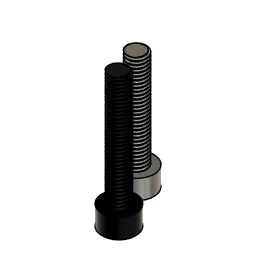
Стенд v5 (Autodesk Fusion 360 archive; units mm, degrees)
design "M6 Hex Screw v3"
Autodesk Fusion 360 part; units mm, degrees
sketch "Sketch1" plane through (0, 0, 0) normal (0, 0, 1) x (1, 0, 0)
  line L0 (0, 0) -> (15, 0) construction
  circle A0 centre (15, 0) radius 5.11
  dimension "d1" = 15
  dimension "d2" = 10.22
  constraint coincident L0.start origin
  constraint horizontal L0
  constraint coincident L0.end A0.centre
  measures "d1" distance of L0.start L0.end
  measures "d2" diameter of A0
extrude "Extrude1" add sketch "Sketch1" along normal blind 6 makes body 1
sketch "Sketch2" plane through (0, 0, 0) normal (0, 0, -1) x (1, 0, 0)
  circle A0 centre (15, 0) radius 5.11
  line L0 (12.43, -1.4838) -> (15, -2.9676)
  line L1 (15, -2.9676) -> (17.57, -1.4838)
  line L2 (17.57, -1.4838) -> (17.57, 1.4838)
  line L3 (17.57, 1.4838) -> (15, 2.9676)
  line L4 (15, 2.9676) -> (12.43, 1.4838)
  line L5 (12.43, 1.4838) -> (12.43, -1.4838)
  point P0 (15, 0)
  dimension "d5" = 2.57
  constraint coincident P0 A0.centre
  constraint vertical L5
  measures "d5" distance of P0 L5
extrude "Extrude2" cut sketch "Sketch2" against normal blind 3 contours L0 L1 L2 L3 L4 L5 bodies 1
fillet "Fillet1" radius 0.2 1 edges at (10.2358, -1.8479, 0) on bodies 1
pattern_circular "C-Pattern1" count 6 over 360 about axis through (0, 0, 1.75) along (0, 0, 1) of bodies 1 makes body 2 at (10.2724, 17.2829, 4.0667) makes body 3 at (-9.8312, 17.5376, 4.0667) makes body 4 at (-20.1036, 0.2547, 4.0667) makes body 5 at (-10.2724, -17.2829, 4.0667) makes body 6 at (9.8312, -17.5376, 4.0667)
sketch "Sketch3" plane through (0, 0, 6) normal (0, 0, 1) x (-1, 0, 0)
  circle A0 centre (-15, 0) radius 5.11
  circle A1 centre (-7.5, -12.9904) radius 5.11
  circle A2 centre (7.5, -12.9904) radius 5.11
  circle A3 centre (15, 0) radius 5.11
  circle A4 centre (7.5, 12.9904) radius 5.11
  circle A5 centre (-7.5, 12.9904) radius 5.11
  circle A6 centre (-15, 0) radius 3
  circle A7 centre (-7.5, -12.9904) radius 3
  circle A8 centre (7.5, -12.9904) radius 3
  circle A9 centre (15, 0) radius 3
  circle A10 centre (7.5, 12.9904) radius 3
  circle A11 centre (-7.5, 12.9904) radius 3
  dimension "d12" = 6
  constraint concentric A0 A6
  constraint concentric A1 A7
  constraint concentric A2 A8
  constraint concentric A3 A9
  constraint concentric A4 A10
  constraint concentric A5 A11
  constraint equal A6 A7
  constraint equal A7 A8
  constraint equal A8 A9
  constraint equal A9 A10
  constraint equal A10 A11
  measures "d12" diameter of A6
extrude "Extrude3" add sketch "Sketch3" along normal blind 10 contours A11 bodies 6
extrude "Extrude4" add sketch "Sketch3" along normal blind 15 contours A6 bodies 1
extrude "Extrude5" add sketch "Sketch3" along normal blind 20 contours A7 bodies 2
extrude "Extrude6" add sketch "Sketch3" along normal blind 25 contours A8 bodies 3
extrude "Extrude7" add sketch "Sketch3" along normal blind 30 contours A9 bodies 4
extrude "Extrude8" add sketch "Sketch3" along normal blind 35 contours A10 bodies 5
thread "Thread1" "ISO Metric profile 6.0 M6x1 6g" major diameter 5.884 minor diameter 4.7435 pitch 1 angle 60 modelled right hand crest width 0.1444 on face at (12.0149, 0.2987, 16) crest through (12.058, 0, 5.75) on face at (-10.4851, 13.2891, 14.3333) crest through (-10.442, 12.9904, 5.75) on face at (-17.9851, 0.2987, 26) crest through (-17.942, 0, 5.75) on face at (-10.4851, -12.6917, 29.3333) crest through (-10.442, -12.9904, 5.75) on face at (4.5037, -12.8408, 12.6667) crest through (4.558, -12.9904, 5.75) on face at (4.5037, 13.1399, 19.3333) crest through (4.558, 12.9904, 5.75) on bodies 1 2 3 4 5 6
hidden bodies 1 2 3 6

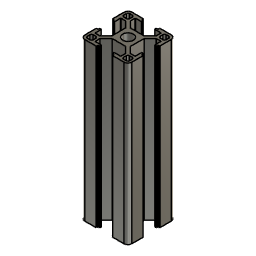
design "profilo alluminio 3030_100mm"
Autodesk Fusion 360 part; units mm, degrees
sketch "Schizzo1" plane through (0, 0, 0) normal (0, 0, 1) x (1, 0, 0)
  circle A0 centre (0, 4) radius 3.4
  line L0 (-12.5, 17.5) -> (-10.7, 17.5) construction
  line L1 (-12.5, 17.5) -> (-10.7, 17.5)
  line L2 (-9.7, 16.5) -> (-9.7, 14.7)
  line L3 (-10.7, 13.7) -> (-12.5, 13.7)
  line L4 (-13.5, 14.7) -> (-13.5, 16.5)
  arc A1 (-9.7, 16.5) -> (-10.7, 17.5) centre (-10.7, 16.5) ccw
  arc A2 (-10.7, 13.7) -> (-9.7, 14.7) centre (-10.7, 14.7) ccw
  arc A3 (-13.5, 14.7) -> (-12.5, 13.7) centre (-12.5, 14.7) ccw
  arc A4 (-12.5, 17.5) -> (-13.5, 16.5) centre (-12.5, 16.5) ccw
  arc A5 (-12.5, 19) -> (-15, 16.5) centre (-12.5, 16.5) ccw
  line L5 (0, 22) -> (0, -17) construction
  line L6 (-9.7, 16.5) -> (-9.7, 19.7766) construction
  line L7 (-12.5, 19) -> (-9.7, 19)
  line L8 (-9.7, 19) -> (-8.2, 19)
  line L9 (-12.8, 12) -> (-12.8, 8.33)
  line L10 (-15, 16.5) -> (-15, 12.2)
  line L11 (-15, 12.2) -> (-15, 9.43)
  line L12 (-13.9, 8.87) -> (-13.9, 8.33)
  line L13 (-13.62, 8.05) -> (-13.08, 8.05)
  line L14 (-12.6, 12.2) -> (-9.816, 12.2)
  line L15 (-9.618, 12.118) -> (-5.882, 8.382)
  line L16 (-8.2, 19) -> (-5.35, 19)
  line L17 (-5.15, 18.8) -> (-5.15, 18.18)
  line L18 (-4.87, 17.9) -> (-4.33, 17.9)
  line L19 (-4.05, 17.62) -> (-4.05, 17.08)
  line L20 (-4.33, 16.8) -> (-7.92, 16.8)
  line L21 (-8.2, 16.52) -> (-8.2, 13.816)
  line L22 (-8.118, 13.618) -> (-4.3003, 9.8003)
  line L23 (0, 4) -> (-21.8842, 3.95)
  line L24 (0, 21) -> (0, -20)
  line L25 (-14.18, 9.15) -> (-14.8, 9.15)
  line L26 (-15, 9.35) -> (-15, 9.43)
  line L27 (-13.9, 8.87) -> (-13.9, 8.95)
  line L28 (-14.1, 9.15) -> (-14.18, 9.15)
  line L29 (-13.9, 8.33) -> (-13.9, 8.25)
  line L30 (-13.7, 8.05) -> (-13.62, 8.05)
  line L31 (-12.8, 8.25) -> (-12.8, 8.33)
  line L32 (-13.08, 8.05) -> (-13, 8.05)
  line L33 (-9.618, 12.118) -> (-9.6414, 12.1414)
  line L34 (-9.7828, 12.2) -> (-9.816, 12.2)
  line L35 (-4.87, 17.9) -> (-4.95, 17.9)
  line L36 (-5.15, 18.18) -> (-5.15, 18.1)
  line L37 (-4.33, 17.9) -> (-4.25, 17.9)
  line L38 (-4.05, 17.7) -> (-4.05, 17.62)
  line L39 (-4.05, 17.08) -> (-4.05, 17)
  line L40 (-4.25, 16.8) -> (-4.33, 16.8)
  line L41 (-7.92, 16.8) -> (-8, 16.8)
  line L42 (-8.2, 16.6) -> (-8.2, 16.52)
  arc A6 (-15, 9.35) -> (-14.8, 9.15) centre (-14.8, 9.35) ccw
  arc A7 (-13.9, 8.95) -> (-14.1, 9.15) centre (-14.1, 8.95) ccw
  arc A8 (-13.9, 8.25) -> (-13.7, 8.05) centre (-13.7, 8.25) ccw
  arc A9 (-13, 8.05) -> (-12.8, 8.25) centre (-13, 8.25) ccw
  arc A10 (-12.6, 12.2) -> (-12.8, 12) centre (-12.6, 12) ccw
  arc A11 (-9.6414, 12.1414) -> (-9.7828, 12.2) centre (-9.7828, 12) ccw
  line L43 (-8.2, 13.816) -> (-8.2, 13.7)
  line L44 (-8.2, 13.7) -> (-8.118, 13.618)
  arc A12 (-5.15, 18.8) -> (-5.35, 19) centre (-5.35, 18.8) ccw
  arc A13 (-5.15, 18.1) -> (-4.95, 17.9) centre (-4.95, 18.1) ccw
  arc A14 (-4.05, 17.7) -> (-4.25, 17.9) centre (-4.25, 17.7) ccw
  arc A15 (-4.25, 16.8) -> (-4.05, 17) centre (-4.25, 17) ccw
  arc A16 (-8, 16.8) -> (-8.2, 16.6) centre (-8, 16.6) ccw
  line L45 (-4.2664, -9.9196) -> (-4.1864, -9.9193)
  line L46 (-8.074, -5.655) -> (-4.2738, -1.8199)
  line L47 (-4.2715, -8.8197) -> (-7.8614, -8.8361)
  line L48 (-3.9902, -9.0984) -> (-3.9906, -9.0184)
  line L49 (-4.1915, -8.8193) -> (-4.2715, -8.8197)
  line L50 (-4.8064, -9.9221) -> (-4.2664, -9.9196)
  line L51 (-12.7633, -4.0584) -> (-12.7801, -0.3884)
  line L52 (-14.9754, -1.4185) -> (-14.975, -1.4985)
  line L53 (-12.7804, -0.3084) -> (-12.7801, -0.3884)
  arc A17 (-14.0763, -1.2144) -> (-13.8772, -1.0135) centre (-14.0772, -1.0144) ccw
  line L54 (-9.6314, -11.0442) -> (-8.1314, -11.0373)
  line L55 (-9.5808, -4.1619) -> (-9.6041, -4.1854)
  line L56 (-9.7453, -4.2446) -> (-9.7784, -4.2448)
  arc A18 (-8.1423, -8.6373) -> (-7.9414, -8.8364) centre (-7.9423, -8.6364) ccw
  line L57 (-4.8064, -9.9221) -> (-4.8864, -9.9225)
  line L58 (-12.4382, -9.557) -> (-10.6382, -9.5488)
  arc A19 (-14.9427, -8.5684) -> (-12.4313, -11.057) centre (-12.4428, -8.557) ccw
  arc A20 (-9.651, -6.7442) -> (-10.6556, -5.7488) centre (-10.651, -6.7488) ccw
  line L59 (-9.5808, -4.1619) -> (-5.8619, -0.4088)
  arc A21 (-12.4555, -5.757) -> (-13.451, -6.7616) centre (-12.451, -6.757) ccw
  line L60 (-13.8776, -0.9335) -> (-13.8772, -1.0135)
  arc A22 (-5.2814, -11.0243) -> (-5.0823, -10.8234) centre (-5.2823, -10.8243) ccw
  arc A23 (-12.7804, -0.3084) -> (-12.9814, -0.1094) centre (-12.9804, -0.3094) ccw
  line L61 (-14.9624, -4.2685) -> (-14.975, -1.4985)
  line L62 (-13.8801, -0.3935) -> (-13.8804, -0.3135)
  line L63 (-12.5624, -4.2575) -> (-9.7784, -4.2448)
  arc A24 (-13.4427, -8.5616) -> (-12.4382, -9.557) centre (-12.4428, -8.557) ccw
  line L64 (-14.0763, -1.2144) -> (-14.1563, -1.2147)
  line L65 (-5.0852, -10.2034) -> (-5.0855, -10.1234)
  line L66 (-8.1551, -5.8533) -> (-8.1556, -5.7374)
  line L67 (-9.6428, -8.5442) -> (-9.6278, -11.8208) construction
  line L68 (-12.4313, -11.057) -> (-9.6314, -11.0442)
  line L69 (-8.1423, -8.6373) -> (-8.1427, -8.5573)
  arc A25 (-9.7453, -4.2446) -> (-9.6041, -4.1854) centre (-9.7462, -4.0446) ccw
  line L70 (-7.8614, -8.8361) -> (-7.9414, -8.8364)
  line L71 (-8.1427, -8.5573) -> (-8.1551, -5.8533)
  line L72 (-10.6556, -5.7488) -> (-12.4555, -5.757)
  line L73 (-13.451, -6.7616) -> (-13.4427, -8.5616)
  arc A26 (-4.8864, -9.9225) -> (-5.0855, -10.1234) centre (-4.8855, -10.1225) ccw
  line L74 (-8.1314, -11.0373) -> (-5.2814, -11.0243)
  line L75 (-8.1556, -5.7374) -> (-8.074, -5.655)
  line L76 (-13.8776, -0.9335) -> (-13.8801, -0.3935)
  line L77 (-13.6014, -0.1122) -> (-13.0614, -0.1097)
  line L78 (-13.0614, -0.1097) -> (-12.9814, -0.1094)
  arc A27 (-10.6382, -9.5488) -> (-9.6428, -8.5442) centre (-10.6428, -8.5488) ccw
  line L79 (-9.6428, -8.5442) -> (-9.651, -6.7442)
  arc A28 (-13.6814, -0.1126) -> (-13.8804, -0.3135) centre (-13.6804, -0.3126) ccw
  line L80 (-14.1563, -1.2147) -> (-14.7763, -1.2176)
  arc A29 (-3.9906, -9.0184) -> (-4.1915, -8.8193) centre (-4.1906, -9.0193) ccw
  line L81 (-14.9427, -8.5684) -> (-14.9624, -4.2685)
  line L82 (-3.9874, -9.7184) -> (-3.9877, -9.6384)
  line L83 (-13.6814, -0.1126) -> (-13.6014, -0.1122)
  arc A30 (-12.7633, -4.0584) -> (-12.5624, -4.2575) centre (-12.5633, -4.0575) ccw
  line L84 (-5.0823, -10.8234) -> (-5.0852, -10.2034)
  arc A31 (-4.1864, -9.9193) -> (-3.9874, -9.7184) centre (-4.1874, -9.7193) ccw
  line L85 (-3.9877, -9.6384) -> (-3.9902, -9.0984)
  arc A32 (-14.7763, -1.2176) -> (-14.9754, -1.4185) centre (-14.7754, -1.4176) ccw
  line L86 (-12.4382, -9.557) -> (-10.6382, -9.5488) construction
  line L87 (-5.882, 8.382) -> (-5.8619, -0.4088)
  line L88 (4.33, 16.8) -> (7.92, 16.8)
  line L89 (4.87, 17.9) -> (4.33, 17.9)
  line L90 (8.074, -5.655) -> (4.2738, -1.8199)
  arc A33 (4.25, 17.9) -> (4.05, 17.7) centre (4.25, 17.7) ccw
  line L91 (4.25, 16.8) -> (4.33, 16.8)
  line L92 (4.05, 17.7) -> (4.05, 17.62)
  arc A34 (13.451, -6.7616) -> (12.4555, -5.757) centre (12.451, -6.757) ccw
  line L93 (5.0852, -10.2034) -> (5.0855, -10.1234)
  line L94 (9.7453, -4.2446) -> (9.7784, -4.2448)
  line L95 (8.1551, -5.8533) -> (8.1556, -5.7374)
  line L96 (9.7, 16.5) -> (9.7, 14.7)
  line L97 (9.6428, -8.5442) -> (9.651, -6.7442)
  line L98 (5.15, 18.8) -> (5.15, 18.18)
  line L99 (14.9427, -8.5684) -> (14.9624, -4.2685)
  line L100 (10.7, 13.7) -> (12.5, 13.7)
  arc A35 (5.35, 19) -> (5.15, 18.8) centre (5.35, 18.8) ccw
  line L101 (7.92, 16.8) -> (8, 16.8)
  line L102 (8.2, 13.816) -> (8.2, 13.7)
  arc A36 (12.5624, -4.2575) -> (12.7633, -4.0584) centre (12.5633, -4.0575) ccw
  arc A37 (10.6556, -5.7488) -> (9.651, -6.7442) centre (10.651, -6.7488) ccw
  line L103 (8.118, 13.618) -> (4.3003, 9.8003)
  line L104 (4.05, 17.08) -> (4.05, 17)
  line L105 (7.8614, -8.8361) -> (7.9414, -8.8364)
  line L106 (12.4382, -9.557) -> (10.6382, -9.5488)
  line L107 (13.6014, -0.1122) -> (13.0614, -0.1097)
  arc A38 (12.9814, -0.1094) -> (12.7804, -0.3084) centre (12.9804, -0.3094) ccw
  line L108 (14.1563, -1.2147) -> (14.7763, -1.2176)
  line L109 (4.8064, -9.9221) -> (4.2664, -9.9196)
  arc A39 (13.8804, -0.3135) -> (13.6814, -0.1126) centre (13.6804, -0.3126) ccw
  line L110 (13.0614, -0.1097) -> (12.9814, -0.1094)
  line L111 (9.7828, 12.2) -> (9.816, 12.2)
  line L112 (14.0763, -1.2144) -> (14.1563, -1.2147)
  arc A40 (7.9414, -8.8364) -> (8.1423, -8.6373) centre (7.9423, -8.6364) ccw
  arc A41 (12.4382, -9.557) -> (13.4427, -8.5616) centre (12.4428, -8.557) ccw
  line L113 (15, 9.35) -> (15, 9.43)
  line L114 (13.8776, -0.9335) -> (13.8772, -1.0135)
  line L115 (9.6428, -8.5442) -> (9.6278, -11.8208) construction
  line L116 (13.5, 14.7) -> (13.5, 16.5)
  line L117 (9.618, 12.118) -> (5.882, 8.382)
  line L118 (13.6814, -0.1126) -> (13.6014, -0.1122)
  line L119 (8.1556, -5.7374) -> (8.074, -5.655)
  arc A42 (14.9754, -1.4185) -> (14.7763, -1.2176) centre (14.7754, -1.4176) ccw
  line L120 (8.2, 16.52) -> (8.2, 13.816)
  arc A43 (13.8772, -1.0135) -> (14.0763, -1.2144) centre (14.0772, -1.0144) ccw
  line L121 (12.8, 12) -> (12.8, 8.33)
  line L122 (3.9877, -9.6384) -> (3.9902, -9.0984)
  arc A44 (3.9874, -9.7184) -> (4.1864, -9.9193) centre (4.1874, -9.7193) ccw
  line L123 (4.1915, -8.8193) -> (4.2715, -8.8197)
  line L124 (5.882, 8.382) -> (5.8619, -0.4088)
  arc A45 (4.1915, -8.8193) -> (3.9906, -9.0184) centre (4.1906, -9.0193) ccw
  line L125 (14.9624, -4.2685) -> (14.975, -1.4985)
  line L126 (9.5808, -4.1619) -> (5.8619, -0.4088)
  arc A46 (4.05, 17) -> (4.25, 16.8) centre (4.25, 17) ccw
  line L127 (4.05, 17.62) -> (4.05, 17.08)
  line L128 (4.33, 17.9) -> (4.25, 17.9)
  line L129 (4.2715, -8.8197) -> (7.8614, -8.8361)
  line L130 (4.8064, -9.9221) -> (4.8864, -9.9225)
  line L131 (13.9, 8.33) -> (13.9, 8.25)
  line L132 (8.2, 13.7) -> (8.118, 13.618)
  line L133 (12.5, 19) -> (9.7, 19)
  arc A47 (5.0855, -10.1234) -> (4.8864, -9.9225) centre (4.8855, -10.1225) ccw
  arc A48 (14.1, 9.15) -> (13.9, 8.95) centre (14.1, 8.95) ccw
  line L134 (12.5624, -4.2575) -> (9.7784, -4.2448)
  line L135 (13.62, 8.05) -> (13.08, 8.05)
  line L136 (8.1427, -8.5573) -> (8.1551, -5.8533)
  line L137 (9.7, 19) -> (8.2, 19)
  line L138 (12.6, 12.2) -> (9.816, 12.2)
  arc A49 (10.7, 17.5) -> (9.7, 16.5) centre (10.7, 16.5) ccw
  line L139 (12.8, 8.25) -> (12.8, 8.33)
  line L140 (10.6556, -5.7488) -> (12.4555, -5.757)
  line L141 (13.08, 8.05) -> (13, 8.05)
  arc A50 (9.6428, -8.5442) -> (10.6382, -9.5488) centre (10.6428, -8.5488) ccw
  arc A51 (9.7828, 12.2) -> (9.6414, 12.1414) centre (9.7828, 12) ccw
  line L142 (13.7, 8.05) -> (13.62, 8.05)
  line L143 (9.7, 16.5) -> (9.7, 19.7766) construction
  arc A52 (15, 16.5) -> (12.5, 19) centre (12.5, 16.5) ccw
  line L144 (8.2, 16.6) -> (8.2, 16.52)
  line L145 (5.0823, -10.8234) -> (5.0852, -10.2034)
  line L146 (13.8776, -0.9335) -> (13.8801, -0.3935)
  arc A53 (13.5, 16.5) -> (12.5, 17.5) centre (12.5, 16.5) ccw
  arc A54 (9.6041, -4.1854) -> (9.7453, -4.2446) centre (9.7462, -4.0446) ccw
  line L147 (13.9, 8.87) -> (13.9, 8.33)
  line L148 (8.1423, -8.6373) -> (8.1427, -8.5573)
  arc A55 (9.7, 14.7) -> (10.7, 13.7) centre (10.7, 14.7) ccw
  arc A56 (12.8, 12) -> (12.6, 12.2) centre (12.6, 12) ccw
  line L149 (9.6314, -11.0442) -> (8.1314, -11.0373)
  arc A57 (12.4313, -11.057) -> (14.9427, -8.5684) centre (12.4428, -8.557) ccw
  line L150 (8.2, 19) -> (5.35, 19)
  arc A58 (4.95, 17.9) -> (5.15, 18.1) centre (4.95, 18.1) ccw
  arc A59 (12.5, 13.7) -> (13.5, 14.7) centre (12.5, 14.7) ccw
  line L151 (9.5808, -4.1619) -> (9.6041, -4.1854)
  line L152 (14.1, 9.15) -> (14.18, 9.15)
  line L153 (9.618, 12.118) -> (9.6414, 12.1414)
  line L154 (12.7804, -0.3084) -> (12.7801, -0.3884)
  line L155 (5.15, 18.18) -> (5.15, 18.1)
  line L156 (13.451, -6.7616) -> (13.4427, -8.5616)
  line L157 (12.4382, -9.557) -> (10.6382, -9.5488) construction
  arc A60 (14.8, 9.15) -> (15, 9.35) centre (14.8, 9.35) ccw
  arc A61 (8.2, 16.6) -> (8, 16.8) centre (8, 16.6) ccw
  line L158 (12.5, 17.5) -> (10.7, 17.5)
  line L159 (13.8801, -0.3935) -> (13.8804, -0.3135)
  line L160 (14.9754, -1.4185) -> (14.975, -1.4985)
  line L161 (4.87, 17.9) -> (4.95, 17.9)
  line L162 (8.1314, -11.0373) -> (5.2814, -11.0243)
  line L163 (14.18, 9.15) -> (14.8, 9.15)
  arc A62 (5.0823, -10.8234) -> (5.2814, -11.0243) centre (5.2823, -10.8243) ccw
  line L164 (12.4313, -11.057) -> (9.6314, -11.0442)
  arc A63 (13.7, 8.05) -> (13.9, 8.25) centre (13.7, 8.25) ccw
  arc A64 (12.8, 8.25) -> (13, 8.05) centre (13, 8.25) ccw
  line L165 (3.9874, -9.7184) -> (3.9877, -9.6384)
  line L166 (15, 12.2) -> (15, 9.43)
  line L167 (13.9, 8.87) -> (13.9, 8.95)
  line L168 (3.9902, -9.0984) -> (3.9906, -9.0184)
  line L169 (15, 16.5) -> (15, 12.2)
  line L170 (12.5, 17.5) -> (10.7, 17.5) construction
  line L171 (12.7633, -4.0584) -> (12.7801, -0.3884)
  line L172 (4.2664, -9.9196) -> (4.1864, -9.9193)
  line L173 (-4.3003, 9.8003) -> (4.3003, 9.8003)
  line L174 (-4.2738, -1.8199) -> (4.2738, -1.8199)
  point P0 (-15, 19)
  point P1 (-13.5, 13.7)
  point P2 (-12.8, 8.05)
  point P3 (-13.9, 9.15)
  point P4 (-13.9, 8.05)
  point P5 (-9.7, 12.2)
  point P6 (-5.15, 19)
  point P7 (-5.15, 17.9)
  point P8 (-4.05, 17.9)
  point P9 (-4.05, 16.8)
  point P10 (-8.2, 16.8)
  point P11 (-15, 9.15)
  point P12 (-13.8813, -0.1135)
  point P13 (-14.9313, -11.0684)
  point P14 (-5.0814, -11.0234)
  point P15 (-13.4555, -5.7616)
  point P16 (-13.8763, -1.2135)
  point P17 (-8.1414, -8.8373)
  point P18 (-12.7814, -0.1084)
  point P19 (-3.9864, -9.9184)
  point P20 (-3.9915, -8.8184)
  point P21 (-14.9763, -1.2185)
  point P22 (-5.0864, -9.9234)
  point P23 (-9.6624, -4.2442)
  point P24 (3.9915, -8.8184)
  point P25 (15, 9.15)
  point P26 (12.8, 8.05)
  point P27 (15, 19)
  point P28 (13.4555, -5.7616)
  point P29 (13.8763, -1.2135)
  point P30 (8.1414, -8.8373)
  point P31 (5.15, 19)
  point P32 (9.6624, -4.2442)
  point P33 (3.9864, -9.9184)
  point P34 (5.0864, -9.9234)
  point P35 (13.9, 9.15)
  point P36 (9.7, 12.2)
  point P37 (4.05, 17.9)
  point P38 (13.8813, -0.1135)
  point P39 (14.9313, -11.0684)
  point P40 (8.2, 16.8)
  point P41 (13.5, 13.7)
  point P42 (14.9763, -1.2185)
  point P43 (13.9, 8.05)
  point P44 (12.7814, -0.1084)
  point P45 (5.0814, -11.0234)
  point P46 (4.05, 16.8)
  point P47 (5.15, 17.9)
  dimension "d1" = 6.8
  dimension "d2" = 1
  dimension "d3" = 1
  dimension "d4" = 2.5
  dimension "d5" = 1.5
  dimension "d6" = 3.05
  dimension "d7" = 1.1
  dimension "d8" = 1.1
  dimension "d9" = 1.1
  dimension "d10" = 4.15
  dimension "d11" = 2.77
  dimension "d12" = 0.28
  dimension "d13" = 0.2
  dimension "d14" = 0.2
  dimension "d15" = 0.2
  constraint horizontal L0
  constraint horizontal L1
  constraint vertical L2
  constraint horizontal L3
  constraint vertical L4
  constraint tangent L2 A1
  constraint tangent L0 A1
  constraint tangent L2 A2
  constraint tangent L3 A2
  constraint equal A1 A2
  constraint coincident P1 L3
  constraint coincident P1 L4
  constraint tangent L3 A3
  constraint tangent L4 A3
  constraint equal A1 A3
  constraint tangent L0 A4
  constraint tangent A1 L6
  constraint coincident L6 L7.end
  constraint tangent A5 L7
  constraint perpendicular L6 L7
  constraint perpendicular L6 L8
  constraint tangent A5 L10
  constraint parallel L8 L16
  constraint perpendicular L16 L17
  constraint perpendicular L17 L18
  constraint perpendicular L16 L19
  constraint perpendicular L19 L20
  constraint perpendicular L16 L21
  constraint coincident A0.centre L23.start
  constraint coincident P4 L12
  constraint coincident P4 L13
  constraint coincident P3 L12
  constraint coincident P2 L13
  constraint coincident P2 L9
  constraint coincident P5 L14
  constraint coincident P5 L15
  constraint coincident P10 L21
  constraint coincident P10 L20
  constraint coincident P9 L20
  constraint coincident P9 L19
  constraint coincident P8 L19
  constraint coincident P8 L18
  constraint coincident P7 L17
  constraint coincident P7 L18
  constraint coincident L5 L24.start
  constraint perpendicular L11 L25
  constraint perpendicular L25 L26
  constraint perpendicular L25 L29
  constraint perpendicular L29 L30
  constraint perpendicular L13 L31
  constraint perpendicular L31 L32
  constraint parallel L14 L34
  constraint parallel L16 L35
  constraint perpendicular L35 L36
  constraint perpendicular L36 L37
  constraint perpendicular L37 L38
  constraint perpendicular L37 L39
  constraint perpendicular L39 L40
  constraint perpendicular L39 L41
  constraint perpendicular L41 L42
  constraint coincident P11 L25
  constraint coincident P11 L26
  constraint tangent L25 A6
  constraint tangent L26 A6
  constraint tangent L27 A7
  constraint tangent L28 A7
  constraint equal A6 A7
  constraint tangent L29 A8
  constraint tangent L30 A8
  constraint equal A6 A8
  constraint tangent L32 A9
  constraint tangent L31 A9
  constraint equal A6 A9
  constraint tangent L9 A10
  constraint tangent L14 A10
  constraint equal A6 A10
  constraint tangent L34 A11
  constraint tangent L33 A11
  constraint parallel L21 L43
  constraint parallel L22 L44
  constraint coincident P6 L16
  constraint coincident P6 L17
  constraint tangent L16 A12
  constraint tangent L17 A12
  constraint tangent L35 A13
  constraint tangent L36 A13
  constraint equal A12 A13
  constraint tangent L37 A14
  constraint tangent L38 A14
  constraint equal A12 A14
  constraint tangent L39 A15
  constraint tangent L40 A15
  constraint equal A12 A15
  constraint tangent L41 A16
  constraint tangent L42 A16
  constraint equal A12 A16
  constraint symmetric P0 L23 P13
  constraint symmetric P1 L23 P15
  constraint symmetric L2.start L23 L67.start
  constraint symmetric L0.end L23 L58.end
  constraint symmetric A1 L23 A27
  constraint symmetric L2.end L23 A20.start
  constraint symmetric L3.start L23 A20.end
  constraint symmetric A2 L23 A20
  constraint symmetric L3.end L23 A21.start
  constraint symmetric L4.start L23 A21.end
  constraint symmetric A3 L23 A21
  constraint symmetric L0.start L23 L58.start
  constraint symmetric L4.end L23 A24.start
  constraint symmetric A4 L23 A24
  constraint symmetric A5.start L23 A19.end
  constraint symmetric A5.end L23 A19.start
  constraint symmetric A5 L23 A19
  constraint symmetric L6.end L23 L67.end
  constraint symmetric L7.end L23 L54.start
  constraint symmetric L8.end L23 L54.end
  constraint symmetric L10.end L23 L61.start
  constraint symmetric P2 L23 P18
  constraint symmetric P3 L23 P16
  constraint symmetric P4 L23 P12
  constraint symmetric P5 L23 P23
  constraint symmetric P6 L23 P14
  constraint symmetric P7 L23 P22
  constraint symmetric P8 L23 P19
  constraint symmetric P9 L23 P20
  constraint symmetric P10 L23 P17
  constraint symmetric L22.end L23 L46.end
  constraint symmetric L23 L11.end L52.end
  constraint symmetric L23 L12.end L62.start
  constraint symmetric L23 L13.start L77.start
  constraint symmetric L23 L25.start L64.end
  constraint symmetric L23 L12.start L60.start
  constraint symmetric L23 L13.end L77.end
  constraint symmetric L23 L9.end L51.end
  constraint symmetric L23 L14.end L56.end
  constraint symmetric L23 L15.start L55.start
  constraint symmetric L23 L15.end L59.end
  constraint symmetric L23 L22.start L46.start
  constraint symmetric L23 L21.end L66.start
  constraint symmetric L23 L21.start L69.end
  constraint symmetric L23 L20.end L47.end
  constraint symmetric L23 L20.start L47.start
  constraint symmetric L23 L19.end L48.start
  constraint symmetric L23 L19.start L82.end
  constraint symmetric L23 L18.end L45.start
  constraint symmetric L23 L17.end L65.start
  constraint symmetric L23 L18.start L50.start
  constraint symmetric L23 P11 P21
  constraint symmetric L23 L25.end L80.end
  constraint symmetric L23 L26.start L52.start
  constraint symmetric L23 A6 A32
  constraint symmetric L23 L27.end A17.end
  constraint symmetric L23 L28.start A17.start
  constraint symmetric L23 A7 A17
  constraint symmetric L23 L29.end L62.end
  constraint symmetric L23 L30.start A28.start
  constraint symmetric L23 A8 A28
  constraint symmetric L23 L32.end A23.end
  constraint symmetric L23 L31.start L53.start
  constraint symmetric L23 A9 A23
  constraint symmetric L23 L9.start L51.start
  constraint symmetric L23 L14.start L63.start
  constraint symmetric L23 A10 A30
  constraint symmetric L23 L34.start L56.start
  constraint symmetric L23 L33.end L55.end
  constraint symmetric L23 A11 A25
  constraint symmetric L23 L43.end L66.end
  constraint symmetric L23 L16.end A22.start
  constraint symmetric L23 L17.start A22.end
  constraint symmetric L23 A12 A22
  constraint symmetric L23 L35.end L57.end
  constraint symmetric L23 L36.end L65.end
  constraint symmetric L23 A13 A26
  constraint symmetric L23 L37.end L45.end
  constraint symmetric L23 L38.start L82.start
  constraint symmetric L23 A14 A31
  constraint symmetric L23 L39.end L48.end
  constraint symmetric L23 L40.start L49.start
  constraint symmetric L23 A15 A29
  constraint symmetric L23 L41.end A18.end
  constraint symmetric L23 L42.start A18.start
  constraint symmetric L23 A16 A18
  constraint symmetric P0 L24 P27
  constraint symmetric P1 L24 P41
  constraint symmetric L2.start L24 L96.start
  constraint symmetric L0.end L24 A49.start
  constraint symmetric A1 L24 A49
  constraint symmetric L2.end L24 L96.end
  constraint symmetric L3.start L24 L100.start
  constraint symmetric A2 L24 A55
  constraint symmetric L3.end L24 L100.end
  constraint symmetric L4.start L24 L116.start
  constraint symmetric A3 L24 A59
  constraint symmetric L0.start L24 A53.end
  constraint symmetric L4.end L24 L116.end
  constraint symmetric A4 L24 A53
  constraint symmetric A5.start L24 L133.start
  constraint symmetric A5.end L24 A52.start
  constraint symmetric A5 L24 A52
  constraint symmetric L6.end L24 L143.end
  constraint symmetric L7.end L24 L133.end
  constraint symmetric L8.end L24 L137.end
  constraint symmetric L10.end L24 L166.start
  constraint symmetric P2 L24 P26
  constraint symmetric P3 L24 P35
  constraint symmetric P4 L24 P43
  constraint symmetric P5 L24 P36
  constraint symmetric P6 L24 P31
  constraint symmetric P7 L24 P47
  constraint symmetric P8 L24 P37
  constraint symmetric P9 L24 P46
  constraint symmetric P10 L24 P40
  constraint symmetric L22.end L24 L103.end
  constraint symmetric L11.end L24 L113.end
  constraint symmetric L12.end L24 L131.start
  constraint symmetric L13.start L24 L135.start
  constraint symmetric L25.start L24 L152.end
  constraint symmetric L12.start L24 L147.start
  constraint symmetric L13.end L24 L135.end
  constraint symmetric L9.end L24 L121.end
  constraint symmetric L14.end L24 L111.end
  constraint symmetric L15.start L24 L117.start
  constraint symmetric L15.end L24 L117.end
  constraint symmetric L22.start L24 L103.start
  constraint symmetric L21.end L24 L102.start
  constraint symmetric L21.start L24 L120.start
  constraint symmetric L20.end L24 L88.end
  constraint symmetric L20.start L24 L88.start
  constraint symmetric L19.end L24 L104.start
  constraint symmetric L19.start L24 L92.end
  constraint symmetric L18.end L24 L89.end
  constraint symmetric L17.end L24 L98.end
  constraint symmetric L18.start L24 L89.start
  constraint symmetric L24 P11 P25
  constraint symmetric L24 L25.end A60.start
  constraint symmetric L24 L26.start L113.start
  constraint symmetric L24 A6 A60
  constraint symmetric L24 L27.end A48.end
  constraint symmetric L24 L28.start A48.start
  constraint symmetric L24 A7 A48
  constraint symmetric L24 L29.end L131.end
  constraint symmetric L24 L30.start L142.start
  constraint symmetric L24 A8 A63
  constraint symmetric L24 L32.end L141.end
  constraint symmetric L24 L31.start L139.start
  constraint symmetric L24 A9 A64
  constraint symmetric L24 L9.start L121.start
  constraint symmetric L24 L14.start L138.start
  constraint symmetric L24 A10 A56
  constraint symmetric L24 L34.start L111.start
  constraint symmetric L24 L33.end A51.end
  constraint symmetric L24 A11 A51
  constraint symmetric L24 L43.end L102.end
  constraint symmetric L24 L16.end A35.start
  constraint symmetric L24 L17.start L98.start
  constraint symmetric L24 A12 A35
  constraint symmetric L24 L35.end A58.start
  constraint symmetric L24 L36.end A58.end
  constraint symmetric L24 A13 A58
  constraint symmetric L24 L37.end A33.start
  constraint symmetric L24 L38.start A33.end
  constraint symmetric L24 A14 A33
  constraint symmetric L24 L39.end L104.end
  constraint symmetric L24 L40.start L91.start
  constraint symmetric L24 A15 A46
  constraint symmetric L24 L41.end L101.end
  constraint symmetric L24 L42.start L144.start
  constraint symmetric L24 A16 A61
  constraint symmetric L24 L65.end L93.end
  constraint symmetric L24 L50.start L109.start
  constraint symmetric L24 L48.end A45.end
  constraint symmetric L24 L45.end A44.end
  constraint symmetric L24 A20.start L97.end
  constraint symmetric L24 A22.end L145.start
  constraint symmetric L24 L65.start L93.start
  constraint symmetric L24 A22.start L162.end
  constraint symmetric L24 A20.end A37.start
  constraint symmetric L24 L66.end L95.end
  constraint symmetric L24 L77.start L107.start
  constraint symmetric L24 L64.end L108.start
  constraint symmetric L24 L57.end L130.end
  constraint symmetric L24 L60.start L114.start
  constraint symmetric L24 L49.start L123.start
  constraint symmetric L24 L82.start A44.start
  constraint symmetric L24 P12 P38
  constraint symmetric L24 L62.end A39.start
  constraint symmetric L24 L53.start A38.end
  constraint symmetric L24 L51.end L154.end
  constraint symmetric L24 L62.start L146.end
  constraint symmetric L24 A28.start A39.end
  constraint symmetric L24 L47.start L123.end
  constraint symmetric L24 A17.end L114.end
  constraint symmetric L24 A17.start L112.start
  constraint symmetric L24 L52.end L125.end
  constraint symmetric L24 L67.start L97.start
  constraint symmetric L24 L48.start L122.end
  constraint symmetric L24 A23.end A38.start
  constraint symmetric L24 L82.end L122.start
  constraint symmetric L24 L80.end L108.end
  constraint symmetric L24 L77.end L107.end
  constraint symmetric L24 L45.start L109.end
  constraint symmetric L24 L58.end L106.end
  constraint symmetric L24 L52.start A42.start
  constraint symmetric L24 L67.end L115.end
  constraint symmetric L24 P13 P39
  constraint symmetric L24 L51.start A36.end
  constraint symmetric L24 L54.end L149.end
  constraint symmetric L24 A19.start L99.start
  constraint symmetric L24 P14 P45
  constraint symmetric L24 L66.start L95.start
  constraint symmetric L24 L46.start L90.start
  constraint symmetric L24 A18.start A40.end
  constraint symmetric L24 A24.start A41.end
  constraint symmetric L24 L55.start L126.start
  constraint symmetric L24 P15 P28
  constraint symmetric L24 L56.start L94.start
  constraint symmetric L24 A21.end A34.start
  constraint symmetric L24 L69.end L136.start
  constraint symmetric L24 P16 P29
  constraint symmetric L24 P17 P30
  constraint symmetric L24 L54.start L149.start
  constraint symmetric L24 L59.end L124.end
  constraint symmetric L24 L46.end L90.end
  constraint symmetric L24 A19.end A57.start
  constraint symmetric L24 P18 P44
  constraint symmetric L24 L61.start L99.end
  constraint symmetric L24 P19 P33
  constraint symmetric L24 A18.end L105.end
  constraint symmetric L24 L47.end L105.start
  constraint symmetric L24 P20 P24
  constraint symmetric L24 P21 P42
  constraint symmetric L24 P22 P34
  constraint symmetric L24 A21.start A34.end
  constraint symmetric L24 L56.end L94.end
  constraint symmetric L24 L58.start L106.start
  constraint symmetric L24 L63.start A36.start
  constraint symmetric L24 P23 P32
  constraint symmetric L24 L55.end A54.start
  constraint symmetric L24 A17 A43
  constraint symmetric L24 A18 A40
  constraint symmetric L24 A19 A57
  constraint symmetric L24 A20 A37
  constraint symmetric L24 A21 A34
  constraint symmetric L24 A22 A62
  constraint symmetric L24 A23 A38
  constraint symmetric L24 A24 A41
  constraint symmetric L24 A25 A54
  constraint symmetric L24 A26 A47
  constraint symmetric L24 A27 A50
  constraint symmetric L24 A28 A39
  constraint symmetric L24 A29 A45
  constraint symmetric L24 A30 A36
  constraint symmetric L24 A31 A44
  constraint symmetric L24 A32 A42
  measures "d1" diameter of A0
  measures "d2" radius of A1
  measures "d3" radius of A4
  measures "d4" radius of A5
  measures "d5" distance of L7.end L8.end
  measures "d6" distance of L8.end P6
  measures "d7" distance of P6 P7
  measures "d8" distance of P7 P8
  measures "d9" distance of P8 P9
  measures "d10" distance of P9 P10
  measures "d11" distance of L10.end L11.end
  measures "d12" distance of L11.end P11
  measures "d13" radius of A6
  measures "d14" radius of A11
  measures "d15" radius of A12
extrude "Estrusione1" add sketch "Schizzo1" along normal blind 100 contours A0 L24 L88 L89 L90 A33 L91 L92 L93 L94 L95 L98 L99 A35 L101 L102 A36 L103 L104 L105 L107 A38 L108 L109 A39 L110 L111 L112 A40 L113 L114 L117 L118 L119 A42 L120 A43 L121 L122 A44 L123 L124 A45 L125 L126 A46 L127 L128 L129 L130 L131 L132 L133 A47 A48 L134 L135 L136 L137 L138 L139 L141 A51 L142 A52 L144 L145 L146 A54 L147 L148 A56 L149 A57 L150 A58 L151 L152 L153 L154 L155 A60 A61 L159 L160 L161 L162 L163 A62 L164 A63 A64 L165 L166 L167 L168 L169 L171 L172 L173 L174 | A0 A5 L7 L8 L9 L10 L11 L12 L13 L14 L15 L16 L17 L18 L19 L20 L21 L22 L23 L24 L25 L26 L27 L28 L29 L30 L31 L32 L33 L34 L35 L36 L37 L38 L39 L40 L41 L42 A6 A7 A8 A9 A10 A11 L43 L44 A12 A13 A14 A15 A16 L87 L173 | A0 L23 L24 L45 L46 L47 L48 L49 L50 L51 L52 L53 A17 L54 L55 L56 A18 L57 A19 L59 L60 A22 A23 L61 L62 L63 L64 L65 L66 L68 L69 A25 L70 L71 A26 L74 L75 L76 L77 L78 A28 L80 A29 L81 L82 L83 A30 L84 A31 L85 A32 L87 L174

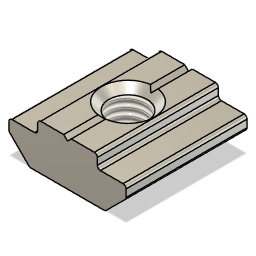
design "Slider T-Nut for 3030 - M6"
Autodesk Fusion 360 part; units mm, degrees
sketch "Sketch1" plane through (0, 0, 0) normal (0, 0, 1) x (1, 0, 0)
  line L0 (2.0362, -0.8565) -> (12.0362, -0.8565)
  line L1 (14.7862, 1.8935) -> (14.7862, 3.4435)
  line L2 (-0.7138, 3.4435) -> (-0.7138, 1.8935)
  line L3 (10.9862, 3.4435) -> (10.9862, 5.1435)
  line L4 (3.0862, 5.1435) -> (3.0862, 3.4435)
  line L5 (-0.7138, 1.8935) -> (2.0362, -0.8565)
  line L6 (7.8157, 5.425) -> (7.8157, -0.8565) construction
  line L7 (14.7862, 1.8935) -> (12.0362, -0.8565)
  line L8 (14.7862, 3.4435) -> (10.9862, 3.4435)
  line L9 (3.0862, 3.4435) -> (-0.7138, 3.4435)
  line L10 (7.0362, 4.6435) -> (7.5362, 5.1435)
  line L11 (7.0362, 4.6435) -> (9.6302, 4.6435) construction
  line L12 (7.0362, 4.6435) -> (6.5362, 5.1435)
  line L13 (7.0362, 4.6435) -> (9.6237, 4.6435) construction
  line L14 (10.9862, 5.1435) -> (7.5362, 5.1435)
  line L15 (6.5362, 5.1435) -> (3.0862, 5.1435)
  dimension "d10" = 3.8
  dimension "d12" = 45
  dimension "d26" = 15.5
  dimension "d27" = 6
  dimension "d28" = 7.9
  dimension "d30" = 7.75
  dimension "d32" = 3.8
  dimension "d33" = 0.5
  dimension "d34" = 1.7
  dimension "d35" = 10
  dimension "d36" = 135
  dimension "d37" = 135
  dimension "d38" = 2.75
  dimension "d39" = 2.75
  constraint horizontal L0
  constraint vertical L1
  constraint horizontal L8
  constraint vertical L2
  constraint vertical L3
  constraint horizontal L14
  constraint vertical L4
  constraint coincident L4.end L8
  constraint coincident L0 L6.end
  constraint perpendicular L0 L6
  constraint collinear L8 L9
  constraint horizontal L11
  constraint perpendicular L10 L12
  constraint horizontal L13
  constraint collinear L14 L15
  constraint equal L1 L2
  constraint equal L5 L7
  measures "d10" distance of L1.end L3.start
  measures "d12" angle of L10 L11
  measures "d26" distance of L1 L2
  measures "d27" distance of L0 L15
  measures "d28" distance of L3 L4
  measures "d30" distance of L2 L10.start
  measures "d32" distance of L2 L4
  measures "d33" distance of L10.start L15
  measures "d34" distance of L9 L15
  measures "d35" distance of L0.start L0.end
  measures "d36" angle of L0 L7
  measures "d37" angle of L0 L5
  measures "d38" horizontal distance of L2.end L0.start
  measures "d39" horizontal distance of L0.end L1.start
extrude "Extrude1" add sketch "Sketch1" along normal blind 16
fillet "Fillet1" radius 0.4 10 edges at (3.0862, 5.1435, 8) (10.9862, 5.1435, 8) (10.9862, 3.4435, 8) (14.7862, 3.4435, 8) (14.7862, 1.8935, 8) (12.0362, -0.8565, 8) (2.0362, -0.8565, 8) (-0.7138, 1.8935, 8) (-0.7138, 3.4435, 8) (3.0862, 3.4435, 8)
hole "Hole1" at (7.0362, 5.1435, 8) direction (0, -1, 0) diameter 5.035 end through all countersink diameter 7 countersink angle 90
thread "Thread1" "ISO Metric profile 6.0 M6x1 6H" thread offset 0 thread depth 10
equation "d30 = ( 15.5 / 2 ) * 1 mm"
equation "d32 = ( ( 15.5 - 7.9 ) / 2 ) * 1 mm"
equation "d36 = 90 deg + 45 deg"
